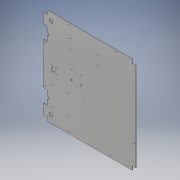
# Autodesk Inventor part: Internal Base Cladding
Saved by Autodesk Inventor 2019 (Build 230136000, 136)
## iProperties
Created: 2018-10-07
Part Number: Internal Base Cladding
Material: Aluminum 6061
Document SubType Name: Sheet Metal
Designer: Ax
Density: 2.7 g/cm^3
Appearance: Aluminum - Dark
Sheet Metal Rule: Default_mm
Mass: 1775.85 g
Surface Area: 4451.61 cm^2
Volume: 657.723 cm^3
Flat Pattern Width: 49 cm
Flat Pattern Length: 51 cm
Flat Pattern Area: 2499 cm^2
Sheet Metal Width: 490.000 mm
Sheet Metal Length: 510.000 mm
Sheet Metal Area: 249900.000 mm^2
Author: Ax
Autodesk Inventor part; units mm, degrees
ref_plane "YZ Plane" through (0, 0, 0) normal (1, 0, 0) x (0, 1, 0)
ref_plane "XZ Plane" through (0, 0, 0) normal (0, 1, 0) x (-1, 0, 0)
ref_plane "XY Plane" through (0, 0, 0) normal (0, 0, 1) x (1, 0, 0)
sketch "Sketch1" plane through (0, 0, 0) normal (0, 1, 0) x (-1, 0, 0)
  line L0 (-245, 255) -> (245, 255)
  line L1 (245, 255) -> (245, -255)
  line L2 (245, -255) -> (-245, -255)
  line L3 (-245, -255) -> (-245, 255)
  line L4 (-245, 255) -> (245, -255) construction
  line L5 (245, 255) -> (-245, -255) construction
  line L6 (225, 255) -> (225, 235)
  line L7 (225, 235) -> (245, 235)
  line L8 (225, -255) -> (225, -235)
  line L9 (225, -235) -> (245, -235)
  line L10 (-225, 255) -> (-225, 235)
  line L11 (-225, 235) -> (-245, 235)
  line L12 (-225, -255) -> (-225, -235)
  line L13 (-225, -235) -> (-245, -235)
  point P0 (0, 0)
  dimension "d0" = 510
  dimension "d1" = 490
  dimension "d2" = 20
  constraints: 28 end point, 8 point on line, 7 equal length, 7 perpendicular, 2 horizontal, 2 midpoint, 2 parallel, 1 vertical
  measures "d0" distance of L0.end L1.end
  measures "d1" distance of L1.end L2.end
  measures "d2" distance of L8.end L8.start
extrude "Extrusion2" add sketch "Sketch1" along normal mid plane 3 contours L0 L6 L7 L1 L9 L8 L2 L12 L13 L3 L11 L10
sketch "Sketch2" plane through (0, -1.5, 0) normal (0, -1, 0) x (1, 0, 0)
  line L0 (235, -245) -> (-235, -245) construction
  line L1 (-235, -245) -> (-235, 245) construction
  line L2 (-235, 245) -> (235, 245) construction
  line L3 (235, 245) -> (235, -245) construction
  line L4 (235, -245) -> (-235, 245) construction
  line L5 (-235, -245) -> (235, 245) construction
  line L6 (-245, 235) -> (-245, -235) construction
  line L7 (225, 255) -> (-225, 255) construction
  circle A0 centre (-235, 98) radius 2.1
  circle A1 centre (-235, -98) radius 2.1
  circle A2 centre (-110, -245) radius 2.1
  circle A3 centre (110, -245) radius 2.1
  circle A4 centre (235, -127.5) radius 2.1
  circle A5 centre (235, 127.5) radius 2.1
  circle A6 centre (135, 245) radius 2.1
  circle A7 centre (-110, 245) radius 2.1
  line L8 (-245, 0) -> (245, 0) construction
  line L9 (-225, 255) -> (225, 255) construction
  line L10 (0, 255) -> (0, -257) construction
  point P0 (0, 0)
  point P1 (0, 0)
  point P2 (0, 0)
  dimension "d7" = 10
  dimension "d8" = 10
  dimension "d9" = 117.5
  dimension "d10" = 100
  dimension "d11" = 4.2
  dimension "d27" = 147
  constraints: 16 end point, 9 point on line, 8 centre point, 7 equal radius, 7 midpoint, 3 symmetric about line, 2 horizontal, 2 parallel, 2 perpendicular
  measures "d7" distance between parallel lines of L1 L6
  measures "d8" distance between parallel lines of L2 L7
  measures "d9" distance of L2.end A5.centre
  measures "d10" distance of L2.end A6.centre
  measures "d11" diameter of A7
  measures "d27" distance of A1.centre L0.end
extrude "Extrusion3" cut sketch "Sketch2" against normal through all
sketch "Sketch3" plane through (0, -1.5, 0) normal (0, -1, 0) x (1, 0, 0)
  line L0 (-205, -15.5) -> (-174, -15.5) construction
  line L1 (-174, -15.5) -> (-174, 15.5) construction
  line L2 (-174, 15.5) -> (-205, 15.5) construction
  line L3 (-205, 15.5) -> (-205, -15.5) construction
  line L4 (-205, -15.5) -> (-174, 15.5) construction
  line L5 (-174, -15.5) -> (-205, 15.5) construction
  line L6 (-245, 235) -> (-245, -235) projected
  line L7 (0, 0) -> (-245, 0) construction
  circle A0 centre (-189.5, 0) radius 11
  circle A1 centre (-205, 15.5) radius 1.7
  circle A2 centre (-174, 15.5) radius 1.7
  circle A3 centre (-174, -15.5) radius 1.7
  circle A4 centre (-205, -15.5) radius 1.7
  point P0 (-189.5, 0)
  dimension "d14" = 40
  dimension "d15" = 22
  dimension "d16" = 31
  dimension "d17" = 3.4
  constraints: 14 end point, 5 centre point, 5 coincident, 4 midpoint, 3 equal radius, 2 parallel, 2 perpendicular, 1 horizontal, 1 point on line
  measures "d14" distance between parallel lines of L3 L6
  measures "d15" diameter of A0
  measures "d16" distance of L0.end L1.end
  measures "d17" diameter of A2
extrude "Extrusion4" cut sketch "Sketch3" against normal through all
sketch "Sketch4" plane through (0, -1.5, 0) normal (0, -1, 0) x (1, 0, 0)
  line L0 (-245, 111.25) -> (-225, 111.25)
  line L1 (-225, 111.25) -> (-225, 181.75)
  line L2 (-225, 181.75) -> (-245, 181.75)
  line L3 (-245, 181.75) -> (-245, 111.25)
  line L4 (-225, 235) -> (-245, 235) projected
  line L5 (-245, 235) -> (-245, -235) projected
  line L6 (-245, 146.5) -> (-216, 146.5) construction
  line L7 (-225, 140.25) -> (-216.5, 140.25)
  line L8 (-216.5, 140.25) -> (-216.5, 152.75)
  line L9 (-216.5, 152.75) -> (-225, 152.75)
  line L10 (-225, 152.75) -> (-225, 140.25)
  point P0 (0, 0)
  dimension "d21" = 70.5
  dimension "d22" = 12.5
  dimension "d23" = 8.5
  dimension "d28" = 20
  dimension "d29" = 88.5
  constraints: 18 end point, 4 parallel, 3 horizontal, 3 point on line, 2 perpendicular, 2 symmetric about line
  measures "d21" distance of L0.end L1.end
  measures "d22" distance of L7.end L8.end
  measures "d23" distance of L8.end L9.end
  measures "d28" distance of L1.end L2.end
  measures "d29" distance of L4.end L6.start
extrude "Extrusion5" cut sketch "Sketch4" against normal through all
mirror "Mirror1" about plane through (0, 0, 0) normal (0, 0, 1) of "Extrusion5"
fillet "Fillet1" radius 1 12 edges at (-225, 0, -111.25) (-216.5, 0, -140.25) (-216.5, 0, -152.75) (-225, 0, -181.75) (-225, 0, -152.75) (-225, 0, -140.25) (-225, 0, 152.75) (-225, 0, 140.25) (-216.5, 0, 152.75) (-225, 0, 181.75) (-216.5, 0, 140.25) (-225, 0, 111.25)
sketch "Sketch6" plane through (0, -1.5, 0) normal (0, -1, 0) x (1, 0, 0)
  line L0 (-105, 185) -> (45, 185) construction
  line L1 (45, 185) -> (45, 135) construction
  line L2 (45, 135) -> (-105, 135) construction
  line L3 (-105, 135) -> (-105, 185) construction
  circle A0 centre (45, 185) radius 2.1
  circle A1 centre (45, 135) radius 2.1
  circle A2 centre (-105, 135) radius 2.1
  circle A3 centre (-105, 185) radius 2.1
  line L4 (225, 255) -> (-225, 255) projected
  line L5 (-245, 235) -> (-245, 181.75) projected
  point P0 (0, 0)
  dimension "d30" = 50
  dimension "d31" = 150
  dimension "d32" = 4.2
  dimension "d33" = 70
  dimension "d34" = 140
  constraints: 8 end point, 4 centre point, 4 coincident, 3 equal radius, 2 parallel, 1 horizontal, 1 perpendicular
  measures "d30" distance of L0.end L1.end
  measures "d31" distance of L0.start L0.end
  measures "d32" diameter of A0
  measures "d33" distance between parallel lines of L4 L0
  measures "d34" distance between parallel lines of L5 L3
hole "Hole1" at (45, -1.5, 185) at (45, -1.5, 135) at (-105, -1.5, 135) at (-105, -1.5, 185) direction (0, 1, 0) diameter 4.2 end through all
sketch "Sketch7" plane through (0, -1.5, 0) normal (0, -1, 0) x (1, 0, 0)
  circle A0 centre (-205, 215) radius 10
  circle A1 centre (-205, -215) radius 10
  line L0 (-205, 215) -> (-205, -215) construction
  line L1 (0, 0) -> (-205, 0) construction
  line L2 (225, 255) -> (-225, 255) construction
  line L3 (-225, -112.25) -> (-225, -139.25) construction
  dimension "d50" = 20
  dimension "d51" = 40
  dimension "d52" = 20
  constraints: 4 end point, 2 centre point, 1 equal radius, 1 horizontal, 1 midpoint, 1 vertical
  measures "d50" diameter of A0
  measures "d51" distance from line of L2 L0.start
  measures "d52" distance between parallel lines of L0 L3
extrude "Cut1" cut sketch "Sketch7" against normal blind 3
sketch "Sketch8" plane through (0, -1.5, 0) normal (0, -1, 0) x (1, 0, 0)
  line L0 (-20, 55) -> (-20, -7) construction
  line L1 (-20, -7) -> (-70, -7) construction
  line L2 (-70, -7) -> (-70, 55) construction
  line L3 (-70, 55) -> (-20, 55) construction
  line L4 (-70, 55) -> (-70, -7) construction
  line L5 (-70, -7) -> (-120, -7) construction
  line L6 (-120, -7) -> (-120, 55) construction
  line L7 (-120, 55) -> (-70, 55) construction
  line L8 (-45, 55) -> (-45, -2.575) construction
  line L9 (-95, 55) -> (-95, -7) construction
  line L10 (225, 255) -> (-225, 255) construction
  circle A0 centre (-45, 47.38) radius 2.1
  line L11 (-45, 1.85) -> (-45, -7) construction
  line L12 (-47.1, 1.85) -> (-47.1, -3.15)
  line L13 (-42.9, -3.15) -> (-42.9, 1.85)
  arc A1 (-42.9, 1.85) -> (-47.1, 1.85) centre (-45, 1.85) ccw
  arc A2 (-47.1, -3.15) -> (-42.9, -3.15) centre (-45, -3.15) ccw
  line L14 (-20, 24) -> (-120, 24) construction
  circle A3 centre (-95, 47.38) radius 2.1
  line L15 (-95, 1.85) -> (-95, -3.15) construction
  line L16 (-97.1, 1.85) -> (-97.1, -3.15)
  line L17 (-92.9, -3.15) -> (-92.9, 1.85)
  arc A4 (-92.9, 1.85) -> (-97.1, 1.85) centre (-95, 1.85) ccw
  arc A5 (-97.1, -3.15) -> (-92.9, -3.15) centre (-95, -3.15) ccw
  line L18 (-245, 111.25) -> (-245, -111.25) projected
  point P0 (0, 0)
  point P1 (-95, -0.65)
  point P2 (-70, 24)
  dimension "d56" = 50
  dimension "d57" = 62
  dimension "d58" = 45.53
  dimension "d59" = 7.62
  dimension "d60" = 5
  dimension "d61" = 4.2
  dimension "d66" = 200
  dimension "d67" = 175
  constraints: 37 end point, 9 midpoint, 8 point on circle, 8 tangent, 7 point on line, 6 centre point, 6 parallel, 3 equal radius, 2 equal length, 2 perpendicular, 2 symmetric about line, 1 horizontal
  measures "d56" distance of L0.end L1.end
  measures "d57" distance of L0.start L0.end
  measures "d58" distance of L11.start A0.centre
  measures "d59" distance from line of L3 A0.centre
  measures "d60" distance of L12.start L12.end
  measures "d61" diameter of A0
  measures "d66" distance between parallel lines of L10 L3
  measures "d67" distance from line of L18 point (-70, 24)
extrude "Cut2" cut sketch "Sketch8" against normal blind 3
sketch "Sketch9" plane through (0, -1.5, 0) normal (0, -1, 0) x (1, 0, 0)
  line L0 (-119.2, -73.2) -> (-195, -73.2) construction
  line L1 (-195, -73.2) -> (-195, -175) construction
  line L2 (-195, -175) -> (-119.2, -175) construction
  line L3 (-119.2, -175) -> (-119.2, -73.2) construction
  line L4 (245, -235) -> (245, 235) construction
  circle A0 centre (-119.2, -73.2) radius 1.7
  circle A1 centre (-119.2, -175) radius 1.7
  circle A2 centre (-195, -175) radius 1.7
  circle A3 centre (-195, -73.2) radius 1.7
  line L5 (-225, -255) -> (225, -255) projected
  line L6 (-245, 111.25) -> (-245, -111.25) projected
  point P0 (0, 0)
  dimension "d68" = 101.8
  dimension "d69" = 75.8
  dimension "d71" = 3.4
  dimension "d74" = 80
  dimension "d75" = 50
  constraints: 8 end point, 4 centre point, 4 coincident, 3 equal radius, 2 parallel, 1 horizontal, 1 perpendicular
  measures "d68" distance of L2.end L0.start
  measures "d69" distance of L1.end L2.end
  measures "d71" diameter of A1
  measures "d74" distance between parallel lines of L5 L2
  measures "d75" distance between parallel lines of L1 L6
extrude "Cut3" cut sketch "Sketch9" against normal blind 3
equation "\"d40\" = Thickness"
equation "\"d54\" = Thickness"
equation "\"d63\" = Thickness"
equation "\"d72\" = Thickness"
equation "\"BendRadius\" = Thickness"
equation "\"BendReliefWidth\" = Thickness"
equation "\"BendReliefDepth\" = 0.5 * Thickness"
equation "\"CornerReliefSize\" = 4 * Thickness"
equation "\"MinimumRemnant\" = 2 * Thickness"
equation "\"TransitionRadius\" = BendRadius"
equation "\"JacobiRadiusSize\" = BendRadius"
equation "\"GapSize\" = Thickness"
equation "\"d53\" = Thickness"
equation "\"Thickness\" = 3"
body "Solid2"
